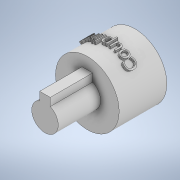
# Autodesk Inventor part: Input Connection
Saved by Autodesk Inventor 2021 (Build 250183000, 183)
## iProperties
Created: 2021-04-10
Part Number: Input Connection
Material: Generic
Document SubType Name: Modeling
Designer: Nabeel Azafer
Density: 1 g/cm^3
Appearance: Default
Mass: 0.862091 g
Surface Area: 7.84277 cm^2
Volume: 0.862091 cm^3
Author: Nabeel Azafer
Autodesk Inventor part; units mm, degrees
ref_plane "YZ Plane" through (0, 0, 0) normal (1, 0, 0) x (0, 1, 0)
ref_plane "XY Plane" through (0, 0, 0) normal (0, 0, 1) x (1, 0, 0)
sketch "Sketch8" plane through (0, 0, 0) normal (0, 0, 1) x (1, 0, 0)
  circle A0 centre (0, 0) radius 6
  dimension "d35" = 12
  constraints: 1 centre point, 1 coincident
  measures "d35" diameter of A0
extrude "Extrusion4" add sketch "Sketch8" along normal blind 7
sketch "Sketch9" plane through (0, 0, 7) normal (0, 0, 1) x (1, 0, 0)
  line L0 (-2.5, 2.5) -> (2.5, 2.5)
  line L1 (2.5, 2.5) -> (2.5, -2.5)
  line L2 (2.5, -2.5) -> (-2.5, -2.5)
  line L3 (-2.5, -2.5) -> (-2.5, 2.5)
  point P0 (0, 0)
  point P1 (0, 0)
  dimension "d38" = 5
  dimension "d39" = 5
  dimension "d40" = 2.5
  dimension "d41" = 2.5
  constraints: 8 end point, 2 parallel, 1 horizontal, 1 perpendicular
  measures "d38" distance of L1.end L2.end
  measures "d39" distance of L2.end L0.start
  measures "d40" distance from line of point (0, 0) L1
  measures "d41" distance from line of point (0, 0) L0
sketch "Sketch10" plane through (0, 0, 0) normal (0, 0, -1) x (-1, 0, 0)
  line L0 (-3, 3) -> (3, 3)
  line L1 (3, 3) -> (3, -3)
  line L2 (3, -3) -> (-3, -3)
  line L3 (-3, -3) -> (-3, 3)
  point P0 (0, 0)
  dimension "d42" = 6
  dimension "d43" = 6
  dimension "d44" = 3
  dimension "d45" = 3
  constraints: 8 end point, 2 parallel, 1 horizontal, 1 perpendicular
  measures "d42" distance of L1.end L2.end
  measures "d43" distance of L2.end L0.start
  measures "d44" distance from line of point (0, 0) L3
  measures "d45" distance from line of point (0, 0) L0
loft "Loft3" cut profiles "Sketch9", "Sketch10"
sketch "Sketch11" plane through (0, 0, 7) normal (0, 0, 1) x (1, 0, 0)
  circle A0 centre (0, 0) radius 6
  constraints: 1 centre point, 1 coincident
extrude "Extrusion5" add sketch "Sketch11" along normal blind 2
sketch "Sketch12" plane through (0, 0, 9) normal (0, 0, 1) x (1, 0, 0)
  circle A0 centre (0, 0) radius 2.5
  dimension "d52" = 5
  constraints: 1 centre point, 1 coincident
  measures "d52" diameter of A0
extrude "Extrusion6" add sketch "Sketch12" along normal blind 8
sketch "Sketch14" plane through (0, 0, 17) normal (0, 0, 1) x (1, 0, 0)
  circle A0 centre (0, 0) radius 2.5 projected
  line L0 (-1, 2.2913) -> (1, 2.2913)
  line L1 (1, 2.2913) -> (1, 3.7913)
  line L2 (1, 3.7913) -> (-1, 3.7913)
  line L3 (-1, 3.7913) -> (-1, 2.2913)
  dimension "d57" = 2
  dimension "d58" = 1.5
  dimension "d59" = 1
  constraints: 8 end point, 2 parallel, 1 horizontal, 1 perpendicular, 2 other
  measures "d57" distance of L2.end L1.end
  measures "d58" distance of L1.end L0.end
  measures "d59" distance from line of point (0, 0) L3
extrude "Extrusion8" add sketch "Sketch14" against normal blind 8 contours L0 A0 | A0 L3 L2 L1 picked at (-0.1703, 2.3433)
ref_plane "Work Plane4" through (0, 7, 0) normal (0, 1, 0) x (-1, 0, 0)
sketch "Sketch16" plane through (0, 7, 0) normal (0, 1, 0) x (-1, 0, 0)
  line L0 (-5.1624, 6.1949) -> (5.8507, 6.1949) construction
  line L1 (5.8507, 6.1949) -> (5.8507, 2.0158) construction
  line L2 (5.8507, 2.0158) -> (-5.1624, 2.0158) construction
  line L3 (-5.1624, 2.0158) -> (-5.1624, 6.1949) construction
  spline S0 degree 2 poles (-4.1786, 4.0701) (-4.3731, 4.0701) (-4.7021, 4.2013) (-4.822, 4.3326) knots 0 0 0 1 2 2 2
  spline S1 degree 2 poles (-4.822, 4.3326) (-4.942, 4.4623) (-5.0732, 4.8513) (-5.0732, 5.1041) knots 0 0 0 1 2 2 2
  spline S2 degree 2 poles (-5.0732, 5.1041) (-5.0732, 5.3553) (-4.9452, 5.7281) (-4.8236, 5.8658) knots 0 0 0 1 2 2 2
  spline S3 degree 2 poles (-4.8236, 5.8658) (-4.7037, 6.0004) (-4.3763, 6.1414) (-4.1737, 6.1414) knots 0 0 0 1 2 2 2
  spline S4 degree 2 poles (-4.1737, 6.1414) (-4.0732, 6.1414) (-3.8966, 6.1122) (-3.822, 6.0895) knots 0 0 0 1 2 2 2
  spline S5 degree 2 poles (-3.822, 6.0895) (-3.7572, 6.0684) (-3.6227, 6.0085) (-3.5562, 5.9728) knots 0 0 0 1 2 2 2
  line L4 (-3.5562, 5.9728) -> (-3.5562, 5.6519)
  line L5 (-3.5562, 5.6519) -> (-3.5773, 5.6519)
  spline S6 degree 2 poles (-3.5773, 5.6519) (-3.613, 5.6843) (-3.7232, 5.7751) (-3.8026, 5.8188) knots 0 0 0 1 2 2 2
  spline S7 degree 2 poles (-3.8026, 5.8188) (-3.8788, 5.861) (-4.0587, 5.9145) (-4.1753, 5.9145) knots 0 0 0 1 2 2 2
  spline S8 degree 2 poles (-4.1753, 5.9145) (-4.3034, 5.9145) (-4.5319, 5.8091) (-4.6178, 5.7086) knots 0 0 0 1 2 2 2
  spline S9 degree 2 poles (-4.6178, 5.7086) (-4.7021, 5.6065) (-4.7961, 5.297) (-4.7961, 5.1041) knots 0 0 0 1 2 2 2
  spline S10 degree 2 poles (-4.7961, 5.1041) (-4.7961, 4.8983) (-4.6972, 4.6017) (-4.6113, 4.4996) knots 0 0 0 1 2 2 2
  spline S11 degree 2 poles (-4.6113, 4.4996) (-4.5271, 4.4007) (-4.3018, 4.3002) (-4.1753, 4.3002) knots 0 0 0 1 2 2 2
  spline S12 degree 2 poles (-4.1753, 4.3002) (-4.0603, 4.3002) (-3.8642, 4.3569) (-3.788, 4.3991) knots 0 0 0 1 2 2 2
  spline S13 degree 2 poles (-3.788, 4.3991) (-3.7151, 4.4412) (-3.6065, 4.5287) (-3.5757, 4.5595) knots 0 0 0 1 2 2 2
  line L6 (-3.5757, 4.5595) -> (-3.5562, 4.5595)
  line L7 (-3.5562, 4.5595) -> (-3.5562, 4.2419)
  spline S14 degree 2 poles (-3.5562, 4.2419) (-3.6227, 4.2111) (-3.7394, 4.1543) (-3.822, 4.1284) knots 0 0 0 1 2 2 2
  spline S15 degree 2 poles (-3.822, 4.1284) (-3.9095, 4.0992) (-4.0587, 4.0701) (-4.1786, 4.0701) knots 0 0 0 1 2 2 2
  spline S16 degree 2 poles (-2.0943, 4.8561) (-2.0943, 4.4769) (-2.459, 4.0636) (-2.7637, 4.0636) knots 0 0 0 1 2 2 2
  spline S17 degree 2 poles (-2.7637, 4.0636) (-3.0765, 4.0636) (-3.4347, 4.4898) (-3.4347, 4.8561) knots 0 0 0 1 2 2 2
  spline S18 degree 2 poles (-3.4347, 4.8561) (-3.4347, 5.2321) (-3.0651, 5.6487) (-2.7637, 5.6487) knots 0 0 0 1 2 2 2
  spline S19 degree 2 poles (-2.7637, 5.6487) (-2.459, 5.6487) (-2.0943, 5.2338) (-2.0943, 4.8561) knots 0 0 0 1 2 2 2
  spline S20 degree 2 poles (-2.3553, 4.8561) (-2.3553, 5.1479) (-2.5676, 5.4315) (-2.7637, 5.4315) knots 0 0 0 1 2 2 2
  spline S21 degree 2 poles (-2.7637, 5.4315) (-2.9598, 5.4315) (-3.1737, 5.1479) (-3.1737, 4.8561) knots 0 0 0 1 2 2 2
  spline S22 degree 2 poles (-3.1737, 4.8561) (-3.1737, 4.5725) (-2.9598, 4.2808) (-2.7637, 4.2808) knots 0 0 0 1 2 2 2
  spline S23 degree 2 poles (-2.7637, 4.2808) (-2.5692, 4.2808) (-2.3553, 4.5676) (-2.3553, 4.8561) knots 0 0 0 1 2 2 2
  line L8 (-0.6681, 4.1057) -> (-0.9209, 4.1057)
  line L9 (-0.9209, 4.1057) -> (-0.9209, 4.271)
  spline S24 degree 2 poles (-0.9209, 4.271) (-1.0376, 4.1689) (-1.2467, 4.0636) (-1.3763, 4.0636) knots 0 0 0 1 2 2 2
  spline S25 degree 2 poles (-1.3763, 4.0636) (-1.4736, 4.0636) (-1.647, 4.1284) (-1.7102, 4.1981) knots 0 0 0 1 2 2 2
  spline S26 degree 2 poles (-1.7102, 4.1981) (-1.775, 4.2678) (-1.8463, 4.4801) (-1.8463, 4.6325) knots 0 0 0 1 2 2 2
  line L10 (-1.8463, 4.6325) -> (-1.8463, 5.6065)
  line L11 (-1.8463, 5.6065) -> (-1.5935, 5.6065)
  line L12 (-1.5935, 5.6065) -> (-1.5935, 4.7508)
  spline S27 degree 2 poles (-1.5935, 4.7508) (-1.5935, 4.6308) (-1.5757, 4.4736) (-1.5449, 4.4153) knots 0 0 0 1 2 2 2
  spline S28 degree 2 poles (-1.5449, 4.4153) (-1.5141, 4.3569) (-1.4087, 4.3035) (-1.3099, 4.3035) knots 0 0 0 1 2 2 2
  spline S29 degree 2 poles (-1.3099, 4.3035) (-1.2175, 4.3035) (-1.0084, 4.4088) (-0.9209, 4.485) knots 0 0 0 1 2 2 2
  line L13 (-0.9209, 4.485) -> (-0.9209, 5.6065)
  line L14 (-0.9209, 5.6065) -> (-0.6681, 5.6065)
  line L15 (-0.6681, 5.6065) -> (-0.6681, 4.1057)
  spline S30 degree 2 poles (0.9559, 4.8966) (0.9559, 4.5206) (0.5977, 4.0765) (0.3238, 4.0765) knots 0 0 0 1 2 2 2
  spline S31 degree 2 poles (0.3238, 4.0765) (0.212, 4.0765) (0.0402, 4.1284) (-0.0489, 4.1819) knots 0 0 0 1 2 2 2
  line L16 (-0.0489, 4.1819) -> (-0.0489, 3.553)
  line L17 (-0.0489, 3.553) -> (-0.3018, 3.553)
  line L18 (-0.3018, 3.553) -> (-0.3018, 5.6065)
  line L19 (-0.3018, 5.6065) -> (-0.0489, 5.6065)
  line L20 (-0.0489, 5.6065) -> (-0.0489, 5.4493)
  spline S32 degree 2 poles (-0.0489, 5.4493) (0.0451, 5.5352) (0.2752, 5.6487) (0.4097, 5.6487) knots 0 0 0 1 2 2 2
  spline S33 degree 2 poles (0.4097, 5.6487) (0.6674, 5.6487) (0.9559, 5.2402) (0.9559, 4.8966) knots 0 0 0 1 2 2 2
  spline S34 degree 2 poles (0.695, 4.8675) (0.695, 5.1252) (0.5313, 5.4088) (0.3482, 5.4088) knots 0 0 0 1 2 2 2
  spline S35 degree 2 poles (0.3482, 5.4088) (0.2412, 5.4088) (0.0402, 5.3132) (-0.0489, 5.2386) knots 0 0 0 1 2 2 2
  line L21 (-0.0489, 5.2386) -> (-0.0489, 4.3861)
  spline S36 degree 2 poles (-0.0489, 4.3861) (0.0499, 4.3391) (0.1909, 4.3035) (0.2817, 4.3035) knots 0 0 0 1 2 2 2
  spline S37 degree 2 poles (0.2817, 4.3035) (0.4778, 4.3035) (0.695, 4.5919) (0.695, 4.8675) knots 0 0 0 1 2 2 2
  line L22 (1.4762, 4.1057) -> (1.2234, 4.1057)
  line L23 (1.2234, 4.1057) -> (1.2234, 6.1949)
  line L24 (1.2234, 6.1949) -> (1.4762, 6.1949)
  line L25 (1.4762, 6.1949) -> (1.4762, 4.1057)
  line L26 (2.105, 4.1057) -> (1.8522, 4.1057)
  line L27 (1.8522, 4.1057) -> (1.8522, 5.6065)
  line L28 (1.8522, 5.6065) -> (2.105, 5.6065)
  line L29 (2.105, 5.6065) -> (2.105, 4.1057)
  line L30 (2.1229, 5.8561) -> (1.836, 5.8561)
  line L31 (1.836, 5.8561) -> (1.836, 6.1187)
  line L32 (1.836, 6.1187) -> (2.1229, 6.1187)
  line L33 (2.1229, 6.1187) -> (2.1229, 5.8561)
  line L34 (3.6545, 4.1057) -> (3.4016, 4.1057)
  line L35 (3.4016, 4.1057) -> (3.4016, 4.9615)
  spline S38 degree 2 poles (3.4016, 4.9615) (3.4016, 5.0652) (3.3822, 5.2435) (3.353, 5.297) knots 0 0 0 1 2 2 2
  spline S39 degree 2 poles (3.353, 5.297) (3.3222, 5.3537) (3.212, 5.4088) (3.118, 5.4088) knots 0 0 0 1 2 2 2
  spline S40 degree 2 poles (3.118, 5.4088) (3.024, 5.4088) (2.8247, 5.3083) (2.729, 5.2273) knots 0 0 0 1 2 2 2
  line L36 (2.729, 5.2273) -> (2.729, 4.1057)
  line L37 (2.729, 4.1057) -> (2.4762, 4.1057)
  line L38 (2.4762, 4.1057) -> (2.4762, 5.6065)
  line L39 (2.4762, 5.6065) -> (2.729, 5.6065)
  line L40 (2.729, 5.6065) -> (2.729, 5.4396)
  spline S41 degree 2 poles (2.729, 5.4396) (2.8425, 5.5417) (3.0613, 5.6487) (3.1845, 5.6487) knots 0 0 0 1 2 2 2
  spline S42 degree 2 poles (3.1845, 5.6487) (3.4049, 5.6487) (3.6545, 5.3569) (3.6545, 5.0798) knots 0 0 0 1 2 2 2
  line L41 (3.6545, 5.0798) -> (3.6545, 4.1057)
  spline S43 degree 2 poles (4.0629, 3.8658) (4.0888, 3.8545) (4.1877, 3.8188) (4.2509, 3.8043) knots 0 0 0 1 2 2 2
  spline S44 degree 2 poles (4.2509, 3.8043) (4.3206, 3.7864) (4.4389, 3.7654) (4.5086, 3.7654) knots 0 0 0 1 2 2 2
  spline S45 degree 2 poles (4.5086, 3.7654) (4.6253, 3.7654) (4.7874, 3.827) (4.8328, 3.8821) knots 0 0 0 1 2 2 2
  spline S46 degree 2 poles (4.8328, 3.8821) (4.8765, 3.9372) (4.9105, 4.0814) (4.9105, 4.1738) knots 0 0 0 1 2 2 2
  line L42 (4.9105, 4.1738) -> (4.9105, 4.3051)
  spline S47 degree 2 poles (4.9105, 4.3051) (4.8084, 4.2159) (4.6123, 4.1317) (4.4648, 4.1317) knots 0 0 0 1 2 2 2
  spline S48 degree 2 poles (4.4648, 4.1317) (4.2088, 4.1317) (3.9057, 4.5125) (3.9057, 4.8707) knots 0 0 0 1 2 2 2
  spline S49 degree 2 poles (3.9057, 4.8707) (3.9057, 5.0571) (4.011, 5.3456) (4.0986, 5.4477) knots 0 0 0 1 2 2 2
  spline S50 degree 2 poles (4.0986, 5.4477) (4.1828, 5.5433) (4.4146, 5.6487) (4.5378, 5.6487) knots 0 0 0 1 2 2 2
  spline S51 degree 2 poles (4.5378, 5.6487) (4.6545, 5.6487) (4.8247, 5.5936) (4.9105, 5.5433) knots 0 0 0 1 2 2 2
  line L43 (4.9105, 5.5433) -> (4.9251, 5.6065)
  line L44 (4.9251, 5.6065) -> (5.1634, 5.6065)
  line L45 (5.1634, 5.6065) -> (5.1634, 4.2775)
  spline S52 degree 2 poles (5.1634, 4.2775) (5.1634, 3.895) (4.8311, 3.5385) (4.4892, 3.5385) knots 0 0 0 1 2 2 2
  spline S53 degree 2 poles (4.4892, 3.5385) (4.3789, 3.5385) (4.1488, 3.5741) (4.0499, 3.6033) knots 0 0 0 1 2 2 2
  line L46 (4.0499, 3.6033) -> (4.0499, 3.8658)
  line L47 (4.0499, 3.8658) -> (4.0629, 3.8658)
  line L48 (4.9105, 4.5125) -> (4.9105, 5.3375)
  spline S54 degree 2 poles (4.9105, 5.3375) (4.8165, 5.3829) (4.6577, 5.4218) (4.5783, 5.4218) knots 0 0 0 1 2 2 2
  spline S55 degree 2 poles (4.5783, 5.4218) (4.387, 5.4218) (4.1666, 5.1398) (4.1666, 4.8756) knots 0 0 0 1 2 2 2
  spline S56 degree 2 poles (4.1666, 4.8756) (4.1666, 4.626) (4.3336, 4.365) (4.5216, 4.365) knots 0 0 0 1 2 2 2
  spline S57 degree 2 poles (4.5216, 4.365) (4.6204, 4.365) (4.8279, 4.4428) (4.9105, 4.5125) knots 0 0 0 1 2 2 2
  point P0 (0, 0)
  constraints: 2 other
emboss "Emboss1" sketch "Sketch16" operation add depth 0.5 direction (0, 1, 0) wrap yes faces at (5.9805, -0.4828, 6)
equation "\"d59\" = 0.5 * d57"
body "Solid4"
